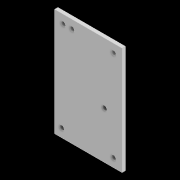
# Autodesk Inventor part: Tapadera_carcasa
Saved by Autodesk Inventor 2020 (Build 240168000, 168)
## iProperties
Created: 2021-12-09
Part Number: Tapadera_carcasa
Material: Generic
Document SubType Name: Modeling
Designer: juan
Density: 1 g/cm^3
Appearance: Default
Author: juan
Autodesk Inventor part; units mm, degrees
ref_plane "YZ Plane" through (0, 0, 0) normal (1, 0, 0) x (0, 1, 0)
ref_plane "XZ Plane" through (0, 0, 0) normal (0, 1, 0) x (-1, 0, 0)
ref_plane "XY Plane" through (0, 0, 0) normal (0, 0, 1) x (1, 0, 0)
sketch "Sketch1" plane through (0, 0, 0) normal (0, 0, 1) x (1, 0, 0)
  line L0 (0, 0) -> (49.5, 0)
  line L1 (49.5, 0) -> (49.5, 79)
  line L2 (49.5, 79) -> (0, 79)
  line L3 (0, 79) -> (0, 0)
  dimension "d0" = 49.5
  dimension "d1" = 79
  constraints: 8 end point, 2 parallel, 1 horizontal, 1 perpendicular
  measures "d0" distance of L2.end L1.end
  measures "d1" distance of L1.end L0.end
extrude "Extrusion1" add sketch "Sketch1" along normal blind 2.5
sketch "Sketch2" plane through (0, 0, 0) normal (0, 0, 1) x (1, 0, 0)
  line L0 (0, 79) -> (0, 0) projected
  line L1 (49.5, 79) -> (0, 79) projected
  point P0 (12.777, 72.735)
  point P1 (36.551, 34.406)
  dimension "d4" = 12.777
  dimension "d5" = 6.265
  dimension "d6" = 38.329
  dimension "d7" = 23.774
  measures "d4" distance from line of L0 point (12.777, 72.735)
  measures "d5" distance from line of L1 point (12.777, 72.735)
  measures "d6" vertical distance of point (12.777, 72.735) point (36.551, 34.406)
  measures "d7" horizontal distance of point (12.777, 72.735) point (36.551, 34.406)
hole "Hole1" at (12.777, 72.735, 0) at (36.551, 34.406, 0) direction (0, 0, 1) diameter 3.3 end through all
sketch "Sketch3" plane through (0, 0, 0) normal (0, 0, 1) x (1, 0, 0)
  line L0 (0, 0) -> (49.5, 0) projected
  line L1 (0, 79) -> (0, 0) projected
  point P0 (5.25, 6.25)
  point P1 (43.25, 6.25)
  point P2 (43.25, 72.75)
  point P3 (6.25, 72.75)
  dimension "d15" = 6.25
  dimension "d16" = 5.25
  dimension "d17" = 38
  dimension "d18" = 72.75
  dimension "d26" = 6.25
  constraints: 2 horizontal alignment, 1 vertical alignment
  measures "d15" distance from line of L0 point (5.25, 6.25)
  measures "d16" distance from line of L1 point (5.25, 6.25)
  measures "d17" distance of point (5.25, 6.25) point (43.25, 6.25)
  measures "d18" distance from line of L0 point (6.25, 72.75)
  measures "d26" distance from line of L1 point (6.25, 72.75)
hole "Hole2" at (5.25, 6.25, 0) at (43.25, 6.25, 0) at (43.25, 72.75, 0) at (6.25, 72.75, 0) direction (0, 0, 1) diameter 3.3 end through all
body "Solid1"
